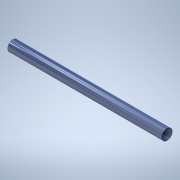
# Autodesk Inventor part: Body Tube
Saved by Autodesk Inventor 2020 (Build 240168000, 168)
## iProperties
Created: 2022-11-08
Part Number: Body Tube
Material: FibreGlass
Document SubType Name: Modeling
Designer: Hp
Density: 1.85 g/cm^3
Appearance: Flaked Satin - Blue
Mass: 1029.3 g
Surface Area: 5573.44 cm^2
Volume: 556.376 cm^3
Author: Hp
Autodesk Inventor part; units mm, degrees
ref_plane "YZ Plane" through (0, 0, 0) normal (1, 0, 0) x (0, 1, 0)
ref_plane "XZ Plane" through (0, 0, 0) normal (0, 1, 0) x (-1, 0, 0)
ref_plane "XY Plane" through (0, 0, 0) normal (0, 0, 1) x (1, 0, 0)
sketch "Sketch1" plane through (0, 0, 0) normal (0, 0, 1) x (1, 0, 0)
  line L0 (0, 0) -> (1150, 0)
  line L1 (1150, 0) -> (1150, 39.5)
  line L2 (1150, 39.5) -> (0, 39.5)
  line L3 (0, 39.5) -> (0, 0)
  line L4 (2, 37.5) -> (1148, 37.5)
  line L5 (1148, 37.5) -> (1150, 37.5)
  line L6 (2, 37.5) -> (0, 37.5)
  dimension "d0" = 1150
  dimension "d1" = 39.5
  dimension "d2" = 2
  constraints: 14 end point, 3 perpendicular, 2 parallel, 2 point on line, 1 horizontal
  measures "d0" distance of L2.end L1.end
  measures "d1" distance of L1.end L0.end
  measures "d2" distance between parallel lines of L2 L4
revolve "Revolution1" add sketch "Sketch1" angle 360 about axis through (0, 0, 0) along (1, 0, 0) contours L3 L2 L1 L5 L4 L6
body "Solid1"
